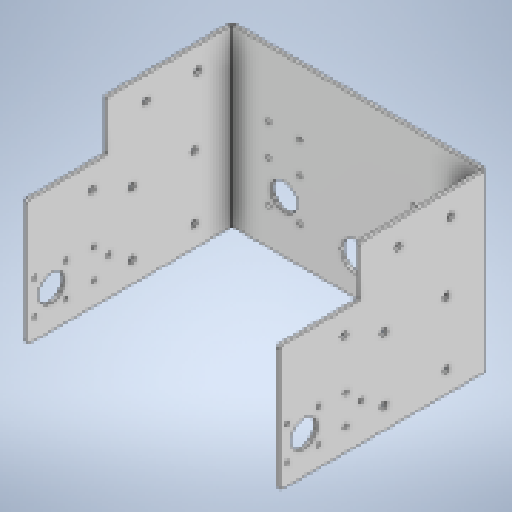
# Autodesk Inventor part: body_main_frame_new
Saved by Autodesk Inventor 2025.2 (Build 292293000, 293)
## iProperties
Created: 2025-05-30
Part Number: body_main_frame_new
Material: Aluminum 6061-AHC
Document SubType Name: Sheet Metal
Designer: chris
Density: 2.7 g/cm^3
Sheet Metal Rule: Default_mm
Appearance: Aluminum - Dark
Author: chris
Autodesk Inventor part; units mm, degrees
ref_plane "YZ Plane" through (0, 0, 0) normal (1, 0, 0) x (0, 1, 0)
ref_plane "XZ Plane" through (0, 0, 0) normal (0, 1, 0) x (-1, 0, 0)
ref_plane "XY Plane" through (0, 0, 0) normal (0, 0, 1) x (1, 0, 0)
sketch "Sketch4" plane through (0, 0, 0) normal (0, 0, 1) x (1, 0, 0)
  line L0 (-60, -42) -> (60, -42)
  line L1 (60, -42) -> (60, 42)
  line L2 (60, 42) -> (-60, 42)
  line L3 (-60, 42) -> (-60, -42)
  line L4 (-60, -42) -> (60, 42) construction
  line L5 (60, -42) -> (-60, 42) construction
  point P0 (0, 0)
  dimension "d13" = 120
  dimension "d14" = 84
  measures "d13" distance of L1.end L2.end
  measures "d14" distance of L0.end L1.end
extrude "Plate3" add sketch "Sketch4" along normal blind 1.5
sketch "Sketch5" plane through (61.5, 42, 0) normal (-1, 0, 0) x (0, -1, 0)
  line L0 (84, 0) -> (0, 0)
  line L1 (0, 0) -> (0, 100)
  line L2 (0, 100) -> (84, 100)
  line L3 (84, 100) -> (84, 0)
  line L4 (40, 5.9925) -> (78.4701, 5.9925)
  line L5 (78.4701, 5.9925) -> (78.4701, 78.464)
  line L6 (78.4701, 78.464) -> (40, 78.464)
  line L7 (40, 78.464) -> (40, 5.9925)
  constraints: 16 end point, 2 parallel, 1 horizontal, 1 perpendicular
edge flange "Flange2" height 100 angle 90 thickness 1.5 bend radius 0.31 thickness toward (-1, 0, 0) relief straight relief width 1.5 relief depth 0.75 corner gap 0.31 corner form 0 edges at (60, 0, 1.5) (-60, 0, 1.5) wall of the first edge with corners at (61.5, -42, 0) (61.5, 42, 0) (61.5, 42, 100) (61.5, -42, 100)
bend "Bend2"
corner "Corner2"
sketch "Sketch6" plane through (-61.5, -42, 100) normal (-1, 0, 0) x (0, 0, 1)
  line L0 (0, 60) -> (-38.5, 60)
  line L1 (-38.5, 60) -> (-38.5, 84)
  line L2 (-38.5, 84) -> (0, 84)
  line L3 (0, 84) -> (0, 60)
  line L4 (0, 84) -> (0, 0) projected
  line L5 (0, 0) -> (-98.19, 0) projected
  line L6 (-98.19, 84) -> (0, 84) projected
  point P0 (-100, 42)
  dimension "d26" = 38.5
  dimension "d27" = 24
  constraints: 8 end point, 2 collinear, 2 parallel, 1 horizontal, 1 perpendicular
  measures "d26" distance of L1.end L2.end
  measures "d27" distance of L2.end L0.start
extrude "Cut1" cut sketch "Sketch6" against normal blind 1.5
sketch "Sketch7" plane through (61.5, -42, 100) normal (1, 0, 0) x (0, 0, -1)
  line L0 (0, 60) -> (38.5, 60)
  line L1 (38.5, 60) -> (38.5, 84)
  line L2 (38.5, 84) -> (0, 84)
  line L3 (0, 84) -> (0, 60)
  line L4 (98.19, 0) -> (0, 0) projected
  line L5 (0, 0) -> (0, 84) projected
  line L6 (0, 84) -> (98.19, 84) projected
  point P0 (100, 42)
  dimension "d30" = 38.5
  dimension "d31" = 24
  constraints: 8 end point, 2 collinear, 2 parallel, 1 horizontal, 1 perpendicular
  measures "d30" distance of L1.end L2.end
  measures "d31" distance of L0.end L1.end
extrude "Cut2" cut sketch "Sketch7" against normal blind 1.5
sketch "Sketch9" plane through (-60, -42, 1.81) normal (1, 0, 0) x (0, 0, -1)
  circle A0 centre (-79.79, 9.93) radius 0.7835 projected
  circle A1 centre (-66.57, 10.93) radius 0.7835 projected
  circle A2 centre (-59.27, 17.93) radius 0.7835 projected
  circle A3 centre (-79.79, 25.93) radius 0.7835 projected
  circle A4 centre (-66.57, 24.93) radius 0.7835 projected
  circle A5 centre (-86.69, 17.93) radius 6 projected
  point P0 (1.81, 42)
hole "Hole1" at (-60, -31.07, 68.38) at (-60, -24.07, 61.08) at (-60, -17.07, 68.38) at (-60, -16.07, 81.6) at (-60, -32.07, 81.6) direction (-1, 0, 0) diameter 2.1 depth 1.5
sketch "Sketch12" plane through (60, -42, 1.81) normal (-1, 0, 0) x (0, 0, 1)
  circle A0 centre (79.79, 25.93) radius 0.7835 projected
  circle A1 centre (79.79, 9.93) radius 0.7835 projected
  circle A2 centre (66.57, 10.93) radius 0.7835 projected
  circle A3 centre (59.27, 17.93) radius 0.7835 projected
  circle A4 centre (66.57, 24.93) radius 0.7835 projected
  point P0 (-1.81, 42)
hole "Hole2" at (60, -32.07, 81.6) at (60, -16.07, 81.6) at (60, -17.07, 68.38) at (60, -24.07, 61.08) at (60, -31.07, 68.38) direction (1, 0, 0) diameter 2.1 depth 1.5
fillet "Corner Round1" radius 1 8 edges at (60.75, -42, 100) (-60.75, -42, 100) (60.75, 18, 100) (60.75, 18, 61.5) (60.75, 42, 61.5) (-60.75, 42, 61.5) (-60.75, 18, 61.5) (-60.75, 18, 100)
sketch "Sketch14" plane through (61.5, -42, 1.81) normal (1, 0, 0) x (0, 0, -1)
  circle A0 centre (-18.19, 10.405) radius 1.55 projected
  circle A1 centre (-48.19, 10.405) radius 1.55 projected
  arc A2 (-55.69, 20) -> (-56.69, 19) centre (-55.69, 19) ccw projected
  line L0 (-55.69, 20) -> (-10.69, 20) projected
  arc A3 (-9.69, 19) -> (-10.69, 20) centre (-10.69, 19) ccw projected
  line L1 (-9.69, 19) -> (-9.69, 1.81) projected
  line L2 (-9.69, 1.81) -> (-56.69, 1.81) projected
  line L3 (-56.69, 19) -> (-56.69, 1.81) projected
  point P0 (1.81, 42)
hole "Hole3" at (61.5, -31.595, 50) at (61.5, -31.595, 20) direction (-1, 0, 0) diameter 3.1 end through all
sketch "Sketch15" plane through (61.5, -42, 1.81) normal (1, 0, 0) x (0, 0, -1)
  circle A0 centre (-18.19, 40.905) radius 1.55 projected
  circle A1 centre (-48.19, 40.905) radius 1.55 projected
  arc A2 (-55.69, 50) -> (-56.69, 49) centre (-55.69, 49) ccw projected
  line L0 (-55.69, 50) -> (-10.69, 50) projected
  arc A3 (-9.69, 49) -> (-10.69, 50) centre (-10.69, 49) ccw projected
  line L1 (-9.69, 49) -> (-9.69, 31.81) projected
  line L2 (-9.69, 31.81) -> (-56.69, 31.81) projected
  line L3 (-56.69, 49) -> (-56.69, 31.81) projected
  circle A4 centre (-18.19, 40.905) radius 1.55 projected
  circle A5 centre (-48.19, 40.905) radius 1.55 projected
  arc A6 (-55.69, 50) -> (-56.69, 49) centre (-55.69, 49) ccw projected
  line L4 (-55.69, 50) -> (-10.69, 50) projected
  arc A7 (-9.69, 49) -> (-10.69, 50) centre (-10.69, 49) ccw projected
  line L5 (-9.69, 49) -> (-9.69, 31.81) projected
  line L6 (-9.69, 31.81) -> (-56.69, 31.81) projected
  line L7 (-56.69, 49) -> (-56.69, 31.81) projected
  point P0 (1.81, 42)
hole "Hole4" at (61.5, -1.095, 50) at (61.5, -1.095, 20) direction (-1, 0, 0) diameter 3.1 end through all
sketch "Sketch16" plane through (61.5, -42, 1.81) normal (1, 0, 0) x (0, 0, -1)
  circle A0 centre (-16.285, 73.095) radius 1.55 projected
  circle A1 centre (-41.285, 73.095) radius 1.55 projected
  arc A2 (-9.785, 64) -> (-8.785, 65) centre (-9.785, 65) ccw projected
  line L0 (-8.785, 65) -> (-8.785, 82.19) projected
  line L1 (-8.785, 82.19) -> (-48.785, 82.19) projected
  line L2 (-48.785, 65) -> (-48.785, 82.19) projected
  arc A3 (-48.785, 65) -> (-47.785, 64) centre (-47.785, 65) ccw projected
  line L3 (-47.785, 64) -> (-9.785, 64) projected
  point P0 (1.81, 42)
hole "Hole5" at (61.5, 31.095, 43.095) at (61.5, 31.095, 18.095) direction (-1, 0, 0) diameter 3.1 end through all
sketch "Sketch17" plane through (61.5, -42, 1.81) normal (1, 0, 0) x (0, 0, -1)
  circle A0 centre (-67.285, 49.095) radius 1.55 projected
  arc A1 (-59.19, 40) -> (-58.19, 41) centre (-59.19, 41) ccw projected
  line L0 (-59.19, 40) -> (-75.38, 40) projected
  arc A2 (-76.38, 41) -> (-75.38, 40) centre (-75.38, 41) ccw projected
  line L1 (-76.38, 41) -> (-76.38, 58.19) projected
  line L2 (-76.38, 58.19) -> (-58.19, 58.19) projected
  line L3 (-58.19, 58.19) -> (-58.19, 41) projected
  point P0 (1.81, 42)
hole "Hole6" at (61.5, 7.095, 69.095) direction (-1, 0, 0) diameter 3.1 end through all
sketch "Sketch20" plane through (-61.5, -42, 1.81) normal (-1, 0, 0) x (0, 0, 1)
  circle A0 centre (59.27, 17.93) radius 0.7835 projected
  circle A1 centre (66.57, 24.93) radius 0.7835 projected
  circle A2 centre (66.57, 10.93) radius 0.7835 projected
  circle A3 centre (79.79, 25.93) radius 0.7835 projected
  circle A4 centre (79.79, 9.93) radius 0.7835 projected
  line L0 (57.87, 11.86) -> (57.87, 24) projected
  line L1 (57.87, 11.86) -> (58.59, 11.86) projected
  arc A5 (60.59, 9.86) -> (58.59, 11.86) centre (58.59, 9.86) ccw projected
  line L2 (60.59, 9.86) -> (60.59, 9.14) projected
  line L3 (92.69, 9.14) -> (60.59, 9.14) projected
  line L4 (92.69, 9.14) -> (92.69, 9.86) projected
  arc A6 (94.69, 11.86) -> (92.69, 9.86) centre (94.69, 9.86) ccw projected
  line L5 (94.69, 11.86) -> (95.41, 11.86) projected
  line L6 (95.41, 24) -> (95.41, 11.86) projected
  line L7 (95.41, 24) -> (94.69, 24) projected
  arc A7 (92.69, 26) -> (94.69, 24) centre (94.69, 26) ccw projected
  line L8 (92.69, 26) -> (92.69, 26.72) projected
  line L9 (60.59, 26.72) -> (92.69, 26.72) projected
  line L10 (60.59, 26.72) -> (60.59, 26) projected
  arc A8 (58.59, 24) -> (60.59, 26) centre (58.59, 26) ccw projected
  line L11 (58.59, 24) -> (57.87, 24) projected
  circle A9 centre (86.69, 17.93) radius 6.4 projected
  point P0 (-1.81, 42)
extrude "Cut4" cut sketch "Sketch20" against normal through all contours A9
sketch "Sketch21" plane through (61.5, -42, 1.81) normal (1, 0, 0) x (0, 0, -1)
  circle A0 centre (-59.27, 17.93) radius 0.7835 projected
  circle A1 centre (-66.57, 10.93) radius 0.7835 projected
  circle A2 centre (-66.57, 24.93) radius 0.7835 projected
  circle A3 centre (-79.79, 9.93) radius 0.7835 projected
  circle A4 centre (-79.79, 25.93) radius 0.7835 projected
  line L0 (-57.87, 24) -> (-57.87, 11.86) projected
  line L1 (-57.87, 24) -> (-58.59, 24) projected
  arc A5 (-60.59, 26) -> (-58.59, 24) centre (-58.59, 26) ccw projected
  line L2 (-60.59, 26) -> (-60.59, 26.72) projected
  line L3 (-92.69, 26.72) -> (-60.59, 26.72) projected
  line L4 (-92.69, 26.72) -> (-92.69, 26) projected
  arc A6 (-94.69, 24) -> (-92.69, 26) centre (-94.69, 26) ccw projected
  line L5 (-94.69, 24) -> (-95.41, 24) projected
  line L6 (-95.41, 11.86) -> (-95.41, 24) projected
  line L7 (-95.41, 11.86) -> (-94.69, 11.86) projected
  arc A7 (-92.69, 9.86) -> (-94.69, 11.86) centre (-94.69, 9.86) ccw projected
  line L8 (-92.69, 9.86) -> (-92.69, 9.14) projected
  line L9 (-60.59, 9.14) -> (-92.69, 9.14) projected
  line L10 (-60.59, 9.14) -> (-60.59, 9.86) projected
  arc A8 (-58.59, 11.86) -> (-60.59, 9.86) centre (-58.59, 9.86) ccw projected
  line L11 (-58.59, 11.86) -> (-57.87, 11.86) projected
  circle A9 centre (-86.69, 17.93) radius 6.4 projected
  point P0 (1.81, 42)
hole "Hole8" at (61.5, -32.14, 96.5) at (61.5, -16, 96.5) direction (-1, 0, 0) diameter 2.1 end through all
sketch "Sketch22" plane through (0, 0, 1.5) normal (0, 0, 1) x (1, 0, 0)
  ellipse E0 centre (-42.882, -24.882) end of major axis (-43.748, -25.748) minor radius 1 (-44, -25.1056) -> (-43.1056, -26) ccw projected
  line L0 (-26.7544, -26) -> (-43.1056, -26) projected
  ellipse E1 centre (-26.978, -24.882) end of major axis (-26.112, -25.748) minor radius 1 (-26.7544, -26) -> (-25.86, -25.1056) ccw projected
  line L1 (-25.86, 11.2056) -> (-25.86, -25.1056) projected
  ellipse E2 centre (-26.978, 10.982) end of major axis (-26.112, 11.848) minor radius 1 (-25.86, 11.2056) -> (-26.7544, 12.1) ccw projected
  line L2 (-43.1056, 12.1) -> (-26.7544, 12.1) projected
  ellipse E3 centre (-42.882, 10.982) end of major axis (-43.748, 11.848) minor radius 1 (-43.1056, 12.1) -> (-44, 11.2056) ccw projected
  line L3 (-44, -25.1056) -> (-44, 11.2056) projected
  circle A0 centre (-27.405, 10.6) radius 0.7835 projected
  circle A1 centre (-42.455, 10.6) radius 0.7835 projected
  circle A2 centre (-27.405, -4.5) radius 0.7835 projected
  circle A3 centre (-42.455, -4.5) radius 0.7835 projected
  circle A4 centre (-27.405, -24.5) radius 0.7835 projected
  circle A5 centre (-42.455, -24.5) radius 0.7835 projected
  circle A6 centre (-34.93, -17) radius 6.4 projected
  ellipse E4 centre (26.978, -24.882) end of major axis (26.112, -25.748) minor radius 1 (25.86, -25.1056) -> (26.7544, -26) ccw projected
  line L4 (43.1056, -26) -> (26.7544, -26) projected
  ellipse E5 centre (42.882, -24.882) end of major axis (43.748, -25.748) minor radius 1 (43.1056, -26) -> (44, -25.1056) ccw projected
  line L5 (44, 11.2056) -> (44, -25.1056) projected
  ellipse E6 centre (42.882, 10.982) end of major axis (43.748, 11.848) minor radius 1 (44, 11.2056) -> (43.1056, 12.1) ccw projected
  line L6 (26.7544, 12.1) -> (43.1056, 12.1) projected
  ellipse E7 centre (26.978, 10.982) end of major axis (26.112, 11.848) minor radius 1 (26.7544, 12.1) -> (25.86, 11.2056) ccw projected
  line L7 (25.86, -25.1056) -> (25.86, 11.2056) projected
  circle A7 centre (42.455, 10.6) radius 0.7835 projected
  circle A8 centre (27.405, 10.6) radius 0.7835 projected
  circle A9 centre (42.455, -4.5) radius 0.7835 projected
  circle A10 centre (27.405, -4.5) radius 0.7835 projected
  circle A11 centre (42.455, -24.5) radius 0.7835 projected
  circle A12 centre (27.405, -24.5) radius 0.7835 projected
  circle A13 centre (34.93, -17) radius 6.4 projected
  point P0 (0, 0)
  constraints: 8 other
hole "Hole9" at (-42.455, -24.5, 1.5) at (-42.455, -4.5, 1.5) at (-42.455, 10.6, 1.5) at (-27.405, 10.6, 1.5) at (-27.405, -4.5, 1.5) at (-27.405, -24.5, 1.5) at (27.405, -24.5, 1.5) at (27.405, -4.5, 1.5) at (27.405, 10.6, 1.5) at (42.455, 10.6, 1.5) at (42.455, -4.5, 1.5) at (42.455, -24.5, 1.5) direction (0, 0, -1) diameter 2.1 depth 1.5 tip angle 118
sketch "Sketch23" plane through (0, 0, 1.5) normal (0, 0, 1) x (1, 0, 0)
  ellipse E0 centre (-42.882, -24.882) end of major axis (-43.748, -25.748) minor radius 1 (-44, -25.1056) -> (-43.1056, -26) ccw projected
  line L0 (-26.7544, -26) -> (-43.1056, -26) projected
  ellipse E1 centre (-26.978, -24.882) end of major axis (-26.112, -25.748) minor radius 1 (-26.7544, -26) -> (-25.86, -25.1056) ccw projected
  line L1 (-25.86, 11.2056) -> (-25.86, -25.1056) projected
  ellipse E2 centre (-26.978, 10.982) end of major axis (-26.112, 11.848) minor radius 1 (-25.86, 11.2056) -> (-26.7544, 12.1) ccw projected
  line L2 (-43.1056, 12.1) -> (-26.7544, 12.1) projected
  ellipse E3 centre (-42.882, 10.982) end of major axis (-43.748, 11.848) minor radius 1 (-43.1056, 12.1) -> (-44, 11.2056) ccw projected
  line L3 (-44, -25.1056) -> (-44, 11.2056) projected
  circle A0 centre (-27.405, 10.6) radius 0.7835 projected
  circle A1 centre (-42.455, 10.6) radius 0.7835 projected
  circle A2 centre (-27.405, -4.5) radius 0.7835 projected
  circle A3 centre (-42.455, -4.5) radius 0.7835 projected
  circle A4 centre (-27.405, -24.5) radius 0.7835 projected
  circle A5 centre (-42.455, -24.5) radius 0.7835 projected
  circle A6 centre (-34.93, -17) radius 6.4 projected
  ellipse E4 centre (26.978, -24.882) end of major axis (26.112, -25.748) minor radius 1 (25.86, -25.1056) -> (26.7544, -26) ccw projected
  line L4 (43.1056, -26) -> (26.7544, -26) projected
  ellipse E5 centre (42.882, -24.882) end of major axis (43.748, -25.748) minor radius 1 (43.1056, -26) -> (44, -25.1056) ccw projected
  line L5 (44, 11.2056) -> (44, -25.1056) projected
  ellipse E6 centre (42.882, 10.982) end of major axis (43.748, 11.848) minor radius 1 (44, 11.2056) -> (43.1056, 12.1) ccw projected
  line L6 (26.7544, 12.1) -> (43.1056, 12.1) projected
  ellipse E7 centre (26.978, 10.982) end of major axis (26.112, 11.848) minor radius 1 (26.7544, 12.1) -> (25.86, 11.2056) ccw projected
  line L7 (25.86, -25.1056) -> (25.86, 11.2056) projected
  circle A7 centre (42.455, 10.6) radius 0.7835 projected
  circle A8 centre (27.405, 10.6) radius 0.7835 projected
  circle A9 centre (42.455, -4.5) radius 0.7835 projected
  circle A10 centre (27.405, -4.5) radius 0.7835 projected
  circle A11 centre (42.455, -24.5) radius 0.7835 projected
  circle A12 centre (27.405, -24.5) radius 0.7835 projected
  circle A13 centre (34.93, -17) radius 6.4 projected
  circle A14 centre (-34.93, -17) radius 6.5
  circle A15 centre (34.93, -17) radius 6.5
  point P0 (0, 0)
  dimension "d106" = 13
  dimension "d107" = 13
  constraints: 2 centre point, 2 coincident, 8 other
  measures "d106" diameter of A14
  measures "d107" diameter of A15
extrude "Cut5" cut sketch "Sketch23" against normal blind 1.5 contours A6 | A13 | A14 | A15
sketch "Sketch24" plane through (0, 0, 0) normal (0, 0, -1) x (-1, 0, 0)
  circle A0 centre (0, -25) radius 7.5
  point P0 (0, 0)
  dimension "d110" = 15
  dimension "d111" = 25
  constraints: 1 centre point
  measures "d110" diameter of A0
  measures "d111" distance of point (0, 0) A0.centre
extrude "Cut6" cut sketch "Sketch24" against normal blind 1.5
equation "\"d28\" = Thickness"
equation "\"d32\" = Thickness"
equation "\"d39\" = Thickness"
equation "\"d48\" = Thickness"
equation "\"d58\" = Thickness"
equation "\"d65\" = Thickness"
equation "\"d79\" = Thickness"
equation "\"d90\" = Thickness"
equation "\"d97\" = Thickness"
equation "\"d104\" = Thickness"
equation "\"d108\" = Thickness"
equation "\"d112\" = Thickness"
equation "\"d15\" = Thickness"
equation "\"d16\" = BendReliefWidth"
equation "\"d17\" = BendReliefDepth"
equation "\"d18\" = MinimumRemnant"
equation "\"d19\" = TransitionRadius"
equation "\"d22\" = BendRadius"
equation "\"d23\" = CornerReliefSize"
equation "\"d24\" = GapSize"
equation "\"d25\" = JacobiRadiusSize"
equation "\"BendReliefWidth\" = Thickness"
equation "\"BendReliefDepth\" = 0.5 * Thickness"
equation "\"CornerReliefSize\" = 4 * Thickness"
equation "\"MinimumRemnant\" = 2 * Thickness"
equation "\"TransitionRadius\" = BendRadius"
equation "\"JacobiRadiusSize\" = BendRadius"
equation "\"GapSize\" = Thickness"
equation "\"Thickness\" = 1.5"
equation "\"BendRadius\" = 0.31"
body "Solid2"
